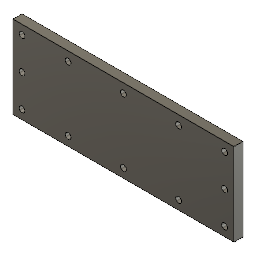
basepanel v5 (Autodesk Fusion 360 design; units mm, degrees)
Autodesk Fusion 360 part; units mm, degrees
sketch "Sketch1" plane through (0, 0, 0) normal (0, 0, 1) x (1, 0, 0)
  line L0 (0, 0) -> (152.4, 0)
  line L1 (152.4, 0) -> (152.4, 57.15)
  line L2 (152.4, 57.15) -> (0, 57.15)
  line L3 (0, 57.15) -> (0, 0)
  circle A0 centre (6.35, 6.35) radius 1.985
  circle A1 centre (146.05, 6.35) radius 1.985
  circle A2 centre (6.35, 50.8) radius 1.985
  circle A3 centre (146.05, 50.8) radius 1.985
  circle A4 centre (6.35, 6.35) radius 1.985
  circle A5 centre (6.35, 28.575) radius 1.985
  circle A6 centre (146.05, 28.575) radius 1.985
  circle A7 centre (76.2, 6.35) radius 1.985
  circle A8 centre (38.1, 6.35) radius 1.985
  circle A9 centre (114.3, 6.35) radius 1.985
  circle A10 centre (38.1, 50.8) radius 1.985
  circle A11 centre (76.2, 50.8) radius 1.985
  circle A12 centre (114.3, 50.8) radius 1.985
  point P0 (6.35, 6.35)
  dimension "d1" = 57.15
  dimension "d2" = 152.4
  dimension "d3" = 3.97
  dimension "d4" = 3.97
  dimension "d5" = 3.97
  dimension "d6" = 3.97
  dimension "d10" = 3.97
  dimension "d11" = 3.97
  dimension "d12" = 3.97
  dimension "d13" = 3.97
  dimension "d14" = 3.97
  dimension "d15" = 3.97
  dimension "d16" = 3.97
  dimension "d17" = 3.97
  dimension "d18" = 3.97
  measures "d1" distance of L0.start L2.end
  measures "d2" distance of L0.start L0.end
  measures "d3" diameter of A0
  measures "d4" diameter of A1
  measures "d5" diameter of A2
  measures "d6" diameter of A3
  measures "d10" diameter of A4
  measures "d11" diameter of A5
  measures "d12" diameter of A6
  measures "d13" diameter of A7
  measures "d14" diameter of A8
  measures "d15" diameter of A9
  measures "d16" diameter of A10
  measures "d17" diameter of A11
  measures "d18" diameter of A12
extrude "Extrude1" add sketch "Sketch1" against normal blind 6.35
